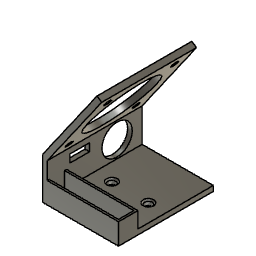
SpeakerBracket v5 (Autodesk Fusion 360 design; units mm, degrees)
Autodesk Fusion 360 part; units mm, degrees
sketch "Sketch1" plane through (0, 0, 0) normal (0, 0, 1) x (1, 0, 0)
  line L0 (0, 0) -> (52, 0)
  line L1 (52, 0) -> (52, 65)
  line L2 (52, 65) -> (0, 65)
  line L3 (0, 65) -> (0, 0)
  circle A0 centre (15, 32.5) radius 2.625
  circle A1 centre (40, 32.5) radius 2.625
  line L4 (0, 65) -> (3.15, 65)
  line L5 (3.15, 65) -> (3.15, 0)
  line L6 (3.15, 0) -> (0, 0)
  line L7 (0, 0) -> (0, 65)
  dimension "d1" = 52
  dimension "d2" = 65
  dimension "d3" = 5.25
  dimension "d4" = 5.25
  dimension "d8" = 25
  dimension "d9" = 3.15
  dimension "d28" = 12
  dimension "d43" = 15
  constraint horizontal L0
  constraint vertical L1
  constraint horizontal L2
  constraint vertical L3
  constraint coincident L0.start L3.end
  constraint horizontal L4
  constraint vertical L5
  constraint horizontal L6
  constraint vertical L7
  constraint coincident L0 L5.end
  measures "d1" distance of L0.start L0.end
  measures "d2" distance of L0.start L2.end
  measures "d3" diameter of A0
  measures "d4" diameter of A1
  measures "d8" distance of A0.centre A1.centre
  measures "d9" distance of L2.end L4.end
  measures "d28" distance of L1 A1.centre
  measures "d43" distance of L3 A0.centre
extrude "Extrude1" add sketch "Sketch1" along normal blind 25 contours L0 L2 L3 L4 L5 L6 L7
extrude "Extrude2" add sketch "Sketch1" against normal blind 3.5
sketch "Sketch2" plane through (0, 0, 0) normal (0, -1, 0) x (1, 0, 0)
  line L0 (3.15, 0) -> (3.15, 25)
  line L1 (3.15, 25) -> (0, 25)
  line L2 (0, 25) -> (0, -3.5)
  line L3 (0, -3.5) -> (52, -3.5)
  line L4 (52, -3.5) -> (52, 0)
  line L5 (52, 0) -> (3.15, 0)
  line L6 (0, 25) -> (3.4667, 22.5726)
  line L7 (0, 25) -> (3.6786, 25) construction
  dimension "d14" = 35
  constraint horizontal L7
  constraint coincident L1.end L2.start
  measures "d14" angle of L6 L7
extrude "Extrude3" cut sketch "Sketch2" against normal through all contours L0 L1 L6
extrude "Extrude4" add 1 faces at (1.05, 21.6667, 24.2648) along direction (0.573576, 0, 0.819152) blind 65
sketch "Sketch3" plane through (-11.7462, 0, 8.2247) normal (-0.819152, 0, 0.573576) x (0, -1, 0)
  line L0 (-65, 20.4788) -> (0, 20.4788)
  line L1 (0, 20.4788) -> (0, 85.4788)
  line L2 (0, 85.4788) -> (-65, 85.4788)
  line L3 (-65, 85.4788) -> (-65, 20.4788)
  circle A0 centre (-9.5, 75.9788) radius 2.5
  circle A1 centre (-32.5, 52.9788) radius 23.75
  line L4 (-32.5, 85.4788) -> (-32.5, 20.4788)
  line L5 (-65, 52.9788) -> (0, 52.9788)
  circle A2 centre (-55.5, 75.9788) radius 2.5
  circle A3 centre (-55.5, 29.9788) radius 2.5
  circle A4 centre (-9.5, 29.9788) radius 2.5
  dimension "d18" = 5
  dimension "d19" = 9.5
  dimension "d20" = 9.5
  dimension "d21" = 47.5
  constraint midpoint L2 L4.start
  constraint midpoint L0 L4.end
  constraint midpoint L3 L5.start
  constraint midpoint L1 L5.end
  constraint midpoint A1.centre L5
  constraint symmetric A0 L4 A2
  constraint symmetric A0 L5 A4
  constraint symmetric L5 A2 A3
  measures "d18" diameter of A0
  measures "d19" distance of L2 A0.centre
  measures "d20" distance of L1 A0.centre
  measures "d21" diameter of A1
extrude "Extrude5" cut sketch "Sketch3" against normal up to surface (3.8454 mm away) contours A1 L4 L5 | A1 L4 L5 | A1 L4 L5 | A1 L4 L5 | A0 | A2 | A3 | A4
chamfer "Chamfer1" distance 1 angle 45 1 edges at (37.5526, 33.4492, 0)
chamfer "Chamfer1" distance 1 angle 45 1 edges at (12.5526, 33.4492, 0)
sketch "Sketch4" plane through (0, 0, 0) normal (-1, 0, 0) x (0, -1, 0)
  line L0 (0, -3.5) -> (0, 25)
  line L1 (0, 25) -> (-65, 25)
  line L2 (-65, 25) -> (-65, -3.5)
  line L3 (-65, -3.5) -> (0, -3.5)
  circle A0 centre (-47.875, 11.3973) radius 10.375
  line L4 (-29, 19) -> (-15.5, 19)
  line L5 (-15.5, 19) -> (-15.5, 13.6)
  line L6 (-15.5, 13.6) -> (-29, 13.6)
  line L7 (-29, 13.6) -> (-29, 19)
  point P0 (-65, 22.7943)
  dimension "d29" = 20.75
  dimension "d30" = 13.5
  dimension "d31" = 5.4
  dimension "d32" = 15.5
  dimension "d34" = 17.125
  dimension "d38" = 6
  dimension "d39" = 11.397
  constraint horizontal L4
  constraint vertical L5
  constraint horizontal L6
  constraint vertical L7
  measures "d29" diameter of A0
  measures "d30" distance of L4.start L4.end
  measures "d31" distance of L4.start L6.end
  measures "d32" distance of L0 L5
  measures "d34" distance of L2 A0.centre
  measures "d38" distance of L1 L4
  measures "d39" vertical distance of A0.centre P0
extrude "Extrude6" cut sketch "Sketch4" against normal through all contours A0 | L4 L5 L6 L7
sketch "Sketch5" plane through (0, 0, 0) normal (0, 0, 1) x (-1, 0, 0)
  circle A0 centre (-40, -32.5) radius 3.625
  line L0 (-3.15, -65) -> (-3.15, 0)
  line L1 (-3.15, 0) -> (-52, 0)
  line L2 (-52, 0) -> (-52, -65)
  line L3 (-52, -65) -> (-3.15, -65)
  circle A1 centre (-15, -32.5) radius 3.625
  line L4 (-3.15, 0) -> (-52, 0)
  line L5 (-52, 0) -> (-52, -13.25)
  line L6 (-52, -13.25) -> (-3.15, -13.25)
  line L7 (-3.15, -13.25) -> (-3.15, 0)
  line L8 (-3.15, -1.375) -> (-50.65, -1.375)
  line L9 (-50.65, -1.375) -> (-50.65, -11.875)
  line L10 (-50.65, -11.875) -> (-3.15, -11.875)
  line L11 (-3.15, -11.875) -> (-3.15, -1.375)
  dimension "d42" = 13.25
  dimension "d44" = 48.85
  dimension "d45" = 47.5
  dimension "d46" = 10.5
  dimension "d47" = 1.375
  constraint horizontal L4
  constraint vertical L5
  constraint horizontal L6
  constraint vertical L7
  constraint coincident L0.end L1.start
  constraint horizontal L8
  constraint vertical L9
  constraint horizontal L10
  constraint vertical L11
  constraint midpoint L7 L11
  measures "d42" distance of L0.end L6.end
  measures "d44" distance of L0.end L1.end
  measures "d45" distance of L8.start L8.end
  measures "d46" distance of L8.start L10.end
  measures "d47" distance of L4 L8
extrude "Extrude7" add sketch "Sketch5" along normal blind 11 contours L0 L1 L2 L4 L5 L6 L7 L8 L9 L10
